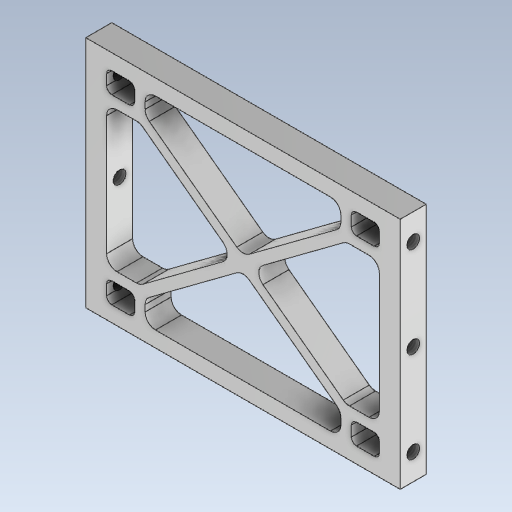
# Autodesk Inventor part: FrontLink_diagonal
Saved by Autodesk Inventor 2020 (Build 240168000, 168)
## iProperties
Part Number: FrontLink_diagonal
Material: アルミニウム 2014-T4
Document SubType Name: Modeling
Designer: MasatoKubotera
Density: 2.8 g/cm^3
Appearance: 滑らか - 淡い灰色
Mass: 13.2133 g
Surface Area: 51.8548 cm^2
Volume: 4.71903 cm^3
Description: A2017 T5
Author: MasatoKubotera
Comments: A2017 T5
Autodesk Inventor part; units mm, degrees
ref_plane "YZ Plane" through (0, 0, 0) normal (1, 0, 0) x (0, 1, 0)
ref_plane "XZ Plane" through (0, 0, 0) normal (0, 1, 0) x (-1, 0, 0)
ref_plane "XY Plane" through (0, 0, 0) normal (0, 0, 1) x (1, 0, 0)
sketch "スケッチ1" plane through (0, 0, 0) normal (1, 0, 0) x (0, 1, 0)
  line L0 (-30.25, 22.5) -> (30.25, 22.5)
  line L1 (30.25, 22.5) -> (30.25, -22.5)
  line L2 (30.25, -22.5) -> (-30.25, -22.5)
  line L3 (-30.25, -22.5) -> (-30.25, 22.5)
  line L4 (-30.25, 22.5) -> (30.25, -22.5) construction
  line L5 (30.25, 22.5) -> (-30.25, -22.5) construction
  line L6 (30.25, 17.5) -> (26.25, 17.5) construction
  line L7 (26.25, 19) -> (26.25, 16) construction
  line L8 (26.25, 16) -> (30.25, 16) construction
  line L9 (26.25, 19) -> (30.25, 19) construction
  line L10 (0, 22.5) -> (0, -22.5)
  line L11 (-30.25, 0) -> (30.25, 0) construction
  line L12 (30.25, -17.5) -> (26.25, -17.5) construction
  line L13 (26.25, -19) -> (26.25, -16) construction
  line L14 (26.25, -16) -> (30.25, -16) construction
  line L15 (26.25, -19) -> (30.25, -19) construction
  line L16 (26.25, 1.5) -> (26.25, -1.5) construction
  line L17 (26.25, -1.5) -> (30.25, -1.5) construction
  line L18 (26.25, 1.5) -> (30.25, 1.5) construction
  line L19 (21.8389, 19.5) -> (25.25, 19.5)
  line L20 (26.25, 18.5) -> (26.25, 16.5)
  line L21 (25.25, 15.5) -> (21.8389, 15.5)
  line L22 (20.8389, 16.5) -> (20.8389, 18.5)
  line L23 (20.8389, 19.5) -> (26.25, 15.5) construction
  line L24 (26.25, 19.5) -> (20.8389, 15.5) construction
  arc A0 (21.8389, 19.5) -> (20.8389, 18.5) centre (21.8389, 18.5) ccw
  arc A1 (20.8389, 16.5) -> (21.8389, 15.5) centre (21.8389, 16.5) ccw
  arc A2 (25.25, 15.5) -> (26.25, 16.5) centre (25.25, 16.5) ccw
  arc A3 (26.25, 18.5) -> (25.25, 19.5) centre (25.25, 18.5) ccw
  line L25 (24.25, 13.5) -> (20.4878, 13.5)
  line L26 (19.2942, 13.1048) -> (3.8331, 1.6048)
  line L27 (24.25, -13.5) -> (20.4878, -13.5)
  line L28 (19.2942, -13.1048) -> (3.8331, -1.6048)
  line L29 (26.25, 11.5) -> (26.25, -11.5)
  line L30 (18.8389, 17.5) -> (18.8389, 16.2637)
  line L31 (18.0325, 14.6589) -> (1.1936, 2.1341)
  line L32 (-18.8389, 17.5) -> (-18.8389, 16.2637)
  line L33 (-18.0325, 14.6589) -> (-1.1936, 2.1341)
  line L34 (-16.8389, 19.5) -> (16.8389, 19.5)
  arc A4 (-16.8389, 19.5) -> (-18.8389, 17.5) centre (-16.8389, 17.5) ccw
  arc A5 (-18.8389, 16.2637) -> (-18.0325, 14.6589) centre (-16.8389, 16.2637) ccw
  arc A6 (-1.1936, 2.1341) -> (1.1936, 2.1341) centre (0, 3.7389) ccw
  arc A7 (18.0325, 14.6589) -> (18.8389, 16.2637) centre (16.8389, 16.2637) ccw
  arc A8 (18.8389, 17.5) -> (16.8389, 19.5) centre (16.8389, 17.5) ccw
  arc A9 (20.4878, 13.5) -> (19.2942, 13.1048) centre (20.4878, 11.5) ccw
  arc A10 (3.8331, 1.6048) -> (3.8331, -1.6048) centre (5.0267, 0) ccw
  arc A11 (19.2942, -13.1048) -> (20.4878, -13.5) centre (20.4878, -11.5) ccw
  arc A12 (24.25, -13.5) -> (26.25, -11.5) centre (24.25, -11.5) ccw
  arc A13 (26.25, 11.5) -> (24.25, 13.5) centre (24.25, 11.5) ccw
  line L35 (18.8389, -17.5) -> (18.8389, -16.2637)
  line L36 (18.0325, -14.6589) -> (1.1936, -2.1341)
  line L37 (-18.8389, -17.5) -> (-18.8389, -16.2637)
  line L38 (-18.0325, -14.6589) -> (-1.1936, -2.1341)
  line L39 (-16.8389, -19.5) -> (16.8389, -19.5)
  arc A14 (-18.8389, -17.5) -> (-16.8389, -19.5) centre (-16.8389, -17.5) ccw
  arc A15 (-18.0325, -14.6589) -> (-18.8389, -16.2637) centre (-16.8389, -16.2637) ccw
  arc A16 (1.1936, -2.1341) -> (-1.1936, -2.1341) centre (0, -3.7389) ccw
  arc A17 (18.8389, -16.2637) -> (18.0325, -14.6589) centre (16.8389, -16.2637) ccw
  arc A18 (16.8389, -19.5) -> (18.8389, -17.5) centre (16.8389, -17.5) ccw
  line L40 (21.8389, -19.5) -> (25.25, -19.5)
  line L41 (26.25, -18.5) -> (26.25, -16.5)
  line L42 (25.25, -15.5) -> (21.8389, -15.5)
  line L43 (20.8389, -16.5) -> (20.8389, -18.5)
  arc A19 (20.8389, -18.5) -> (21.8389, -19.5) centre (21.8389, -18.5) ccw
  arc A20 (21.8389, -15.5) -> (20.8389, -16.5) centre (21.8389, -16.5) ccw
  arc A21 (26.25, -16.5) -> (25.25, -15.5) centre (25.25, -16.5) ccw
  arc A22 (25.25, -19.5) -> (26.25, -18.5) centre (25.25, -18.5) ccw
  point P0 (0, 0)
  point P1 (26.25, 0)
  point P2 (23.5444, 17.5)
  point P3 (26.25, 13.5)
  point P4 (19.8256, 13.5)
  point P5 (1.6756, 0)
  point P6 (26.25, -13.5)
  point P7 (19.8256, -13.5)
  point P8 (18.8389, 19.5)
  point P9 (18.8389, 15.2587)
  point P10 (0, 1.2463)
  point P11 (-18.8389, 19.5)
  point P12 (-18.8389, 15.2587)
  point P13 (0, -19.5)
  point P14 (0, 19.5)
  point P15 (0, 1.7389)
  point P16 (0, -1.7389)
  dimension "d0" = 60.5
  dimension "d1" = 45
  dimension "d2" = 4
  dimension "d3" = 3
  dimension "d5" = 3
  dimension "d6" = 35
  dimension "d8" = 1
  dimension "d10" = 3
  dimension "d11" = 2
  dimension "d12" = 2
  dimension "d13" = 2
  dimension "d14" = 2
  constraints: 88 end point, 46 point on circle, 37 point on line, 37 symmetric about line, 28 tangent, 23 centre point, 12 equal radius, 11 midpoint, 6 parallel, 6 perpendicular, 5 horizontal, 4 collinear, 4 vertical, 10 other
  measures "d0" distance of L0.start L0.end
  measures "d1" distance of L0.end L1.end
  measures "d2" distance of L6.end L6.start
  measures "d3" distance of L7.start L7.end
  measures "d5" distance of L18.start L17.start
  measures "d6" distance of L12.start L6.start
  measures "d8" radius of A0
  measures "d10" distance between parallel lines of L0 L19
  measures "d11" distance between parallel lines of L25 L21
  measures "d12" distance between parallel lines of L26 L31
  measures "d13" distance between parallel lines of L30 L22
  measures "d14" radius of A4
extrude "押し出し1" add sketch "スケッチ1" along normal blind 5 contours L0 L1 L2 L10 L39 A18 L35 A17 L36 A16 A6 L31 A7 L30 A8 L34
sketch "スケッチ2" plane through (0, 30.25, 22.5) normal (0, 1, 0) x (1, 0, 0)
  line L0 (5, 45) -> (5, 0) projected
  line L1 (5, 5) -> (0, 5) construction
  line L2 (0, 45) -> (0, 0) projected
  line L3 (5, 40) -> (0, 40) construction
  line L4 (5, 5) -> (0, 5) construction
  line L5 (5, 22.5) -> (0, 22.5) construction
  point P0 (2.5, 22.5)
  point P1 (2.5, 5)
  point P2 (2.5, 40)
  point P3 (2.5, 40)
  point P4 (2.5, 5)
  point P5 (2.5, 22.5)
  constraints: 8 end point, 6 midpoint, 4 point on line, 3 coincident, 3 horizontal
hole "穴1" at (2.5, 30.25, -17.5) at (2.5, 30.25, 0) at (2.5, 30.25, 17.5) direction (0, -1, 0) diameter 2.459 depth 5 thread size "M3x0.5" class "6H" standard "ISO Metric profile"
mirror "ミラー1" about plane through (0, 0, 22.5) normal (0, -1, 0)
equation "\"d13\" = d11"
